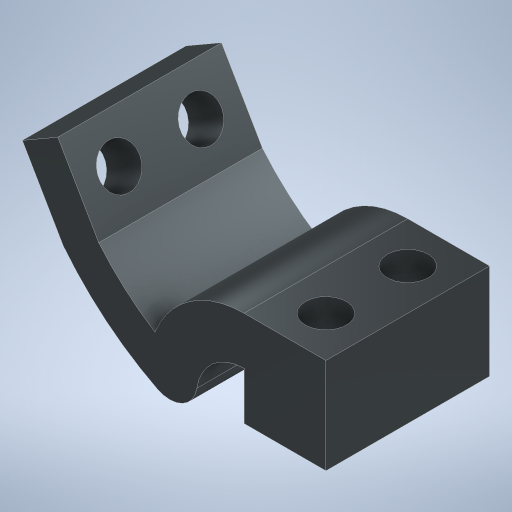
# Autodesk Inventor part: acople
Saved by Autodesk Inventor 2024 (Build 280153000, 153)
## iProperties
Created: 2023-12-04
Part Number: acople
Material: Iron, Ductile
Document SubType Name: Modeling
Designer: Juan_Daleman
Density: 7.15 g/cm^3
Appearance: Iron Gray
Author: Juan_Daleman
Autodesk Inventor part; units mm, degrees
ref_plane "YZ Plane" through (0, 0, 0) normal (1, 0, 0) x (0, 1, 0)
ref_plane "XZ Plane" through (0, 0, 0) normal (0, 1, 0) x (-1, 0, 0)
ref_plane "XY Plane" through (0, 0, 0) normal (0, 0, 1) x (1, 0, 0)
sketch "Sketch1" plane through (0, 0, 0) normal (0, 0, 1) x (1, 0, 0)
  circle A0 centre (0, 0) radius 17.5
  line L0 (-15.1554, -8.75) -> (-13.6554, -11.3481)
  line L1 (-15.1554, -8.75) -> (-16.6554, -6.1519)
  line L2 (-16.6554, -6.1519) -> (-19.2535, -7.6519)
  line L3 (-19.2535, -7.6519) -> (-16.2535, -12.8481)
  line L4 (0, 0) -> (0, -17.5)
  line L5 (0, 0) -> (15.1554, -8.75)
  line L6 (0, 0) -> (17.5, 0) construction
  line L7 (0, 0) -> (17.5, 0) construction
  line L8 (0, 17.5) -> (0, -17.5)
  line L9 (-15.1554, -8.75) -> (0, 0)
  line L10 (0, -17.5) -> (3, -17.5)
  line L11 (3, -17.5) -> (3, -20.5)
  line L12 (-3, -17.5) -> (0, -17.5)
  arc A1 (-16.2535, -12.8481) -> (-3, -20.5) centre (0, 0) ccw
  line L13 (-3, -17.5) -> (-3, -14)
  line L14 (-3, -10.5) -> (3, -10.5)
  line L15 (3, -10.5) -> (3, -17.5)
  arc A2 (-3, -10.5) -> (-9.5308, -14.9804) centre (-3, -17.5) ccw
  arc A3 (-3, -14) -> (-5.4652, -19.9845) centre (-3, -17.5) ccw
  arc A4 (-13.6554, -11.3481) -> (-9.5308, -14.9804) centre (0, 0) ccw
  arc A5 (-6.3746, -16.5715) -> (-3, -17.5) centre (0, 0) ccw
  point P0 (0, -10.5)
  point P1 (-3, -17.2409)
  point P2 (3, -17.2409)
  dimension "d0" = 35
  dimension "d1" = 3
  dimension "d2" = 3
  dimension "d3" = 3
  dimension "d4" = 330
  dimension "d6" = 35
  dimension "d8" = 3
  dimension "d9" = 3
  dimension "d10" = 6
  dimension "d11" = 3
  dimension "d29" = 7
  dimension "d30" = 6
  constraints: 32 end point, 12 point on circle, 5 centre point, 5 perpendicular, 4 coincident, 4 point on line, 3 horizontal, 2 vertical, 1 equal length, 1 midpoint, 3 other
  measures "d1" distance of L0.start L0.end
  measures "d2" distance of L0.end L3.end
  measures "d3" distance of L0.start L1.end
  measures "d6" distance of L8.start L8.end
  measures "d8" distance of L4.end L10.end
  measures "d9" distance of L10.end L11.end
  measures "d10" distance of L11.end A1.end
  measures "d11" distance of A1.end L12.start
  measures "d29" distance of L12.start L14.start
  measures "d30" distance of L14.start L14.end
extrude "Extrusion1" add sketch "Sketch1" along normal blind 12 contours L0 A4 A2 A0 A3 A1 L3 L2 L1 | L15 L10 A0 | A0 L4 L14 L15 | A2 L14 L4 A0 L13 A3 | L12 L13 A0
sketch "Sketch2" plane through (-16.6554, -6.1519, 12) normal (0.866, 0.5, 0) x (0, 0, -1)
  line L0 (0, 0) -> (0, -3)
  line L1 (12, -6) -> (0, -6) projected
  line L2 (0, -3) -> (12, -3)
  line L3 (0, -3) -> (3, -3)
  line L4 (3, -3) -> (9, -3)
  circle A0 centre (3, -3) radius 1.5
  circle A1 centre (9, -3) radius 1.5
  dimension "d14" = 3
  dimension "d15" = 3
  dimension "d16" = 6
  dimension "d17" = 3
  dimension "d18" = 3
  constraints: 8 end point, 2 centre point, 2 coincident, 2 perpendicular, 2 point on line
  measures "d14" distance of L0.start L0.end
  measures "d15" distance of L0.end L3.end
  measures "d16" distance of L3.end L4.end
  measures "d17" diameter of A0
  measures "d18" diameter of A1
extrude "Extrusion2" cut sketch "Sketch2" against normal blind 12
sketch "Sketch3" plane through (-3, -17.5, 0) normal (0, -1, 0) x (1, 0, 0)
  line L0 (6, 12) -> (0, 12) projected
  line L1 (3, 0) -> (3, 3)
  line L2 (3, 3) -> (3, 9)
  circle A0 centre (3, 3) radius 1.5
  circle A1 centre (3, 9) radius 1.5
  dimension "d23" = 3
  dimension "d24" = 6
  dimension "d25" = 3
  dimension "d26" = 3
  constraints: 4 end point, 2 centre point, 2 coincident, 1 point on line, 1 vertical
  measures "d23" distance of L1.start L1.end
  measures "d24" distance of L1.end L2.end
  measures "d25" diameter of A0
  measures "d26" diameter of A1
extrude "Extrusion3" cut sketch "Sketch3" against normal blind 12
fillet "Fillet1" radius 2 1 edges at (-5.4652, -19.9845, 6)
body "Solid1"
